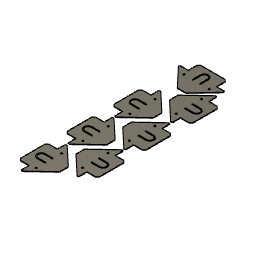
MagneticClampHanger v1 (Autodesk Fusion 360 design; units mm, degrees)
Autodesk Fusion 360 part; units mm, degrees
sketch "Sketch1" plane through (0, 0, 0) normal (0, 1, 0) x (1, 0, 0)
  line L0 (0, 0) -> (92.202, 0)
  line L1 (0, 0) -> (0, 34.29)
  line L2 (92.202, 0) -> (92.202, 34.29)
  line L3 (0, 34.29) -> (-31.75, 34.29)
  line L4 (92.202, 34.29) -> (123.952, 34.29)
  line L5 (46.101, 0) -> (46.101, 101.981) construction
  line L6 (46.101, 101.981) -> (60.071, 101.981) construction
  line L7 (60.071, 101.981) -> (123.952, 34.29)
  line L8 (60.071, 101.981) -> (32.131, 101.981)
  line L9 (32.131, 101.981) -> (-31.75, 34.29)
  line L10 (46.101, 0) -> (46.101, 31.75) construction
  line L11 (46.101, 101.981) -> (46.101, 60.833) construction
  line L12 (46.101, 60.833) -> (46.101, 46.2915) construction
  circle A0 centre (46.101, 46.2915) radius 14.5415 construction
  line L13 (-6.604, -6.604) -> (-6.604, 27.686)
  line L14 (-6.604, 27.686) -> (-47.0627, 27.686)
  line L15 (29.2829, 108.585) -> (-47.0627, 27.686)
  line L16 (62.9191, 108.585) -> (29.2829, 108.585)
  line L17 (62.9191, 108.585) -> (139.2647, 27.686)
  line L18 (98.806, 27.686) -> (139.2647, 27.686)
  line L19 (98.806, -6.604) -> (98.806, 27.686)
  line L20 (-6.604, -6.604) -> (98.806, -6.604)
  line L21 (58.6943, 53.5623) -> (33.5077, 53.5623) construction
  line L22 (33.5077, 53.5623) -> (35.0952, 53.5623)
  line L23 (58.6943, 53.5623) -> (57.1068, 53.5623)
  line L24 (35.0952, 53.5623) -> (35.0952, 28.1623)
  line L25 (57.1068, 53.5623) -> (57.1068, 28.1623)
  arc A1 (35.0952, 28.1623) -> (57.1068, 28.1623) centre (46.101, 28.1623) ccw
  line L26 (33.5077, 51.9748) -> (33.5077, 28.1623)
  arc A2 (33.5077, 28.1623) -> (58.6943, 28.1623) centre (46.101, 28.1623) ccw
  line L27 (58.6943, 51.9748) -> (58.6943, 28.1623)
  line L28 (33.5077, 51.9748) -> (33.5077, 53.5623)
  line L29 (58.6943, 51.9748) -> (58.6943, 53.5623)
  dimension "d1" = 92.202
  dimension "d2" = 34.29
  dimension "d3" = 34.29
  dimension "d4" = 31.75
  dimension "d5" = 31.75
  dimension "d6" = 101.981
  dimension "d7" = 13.97
  dimension "d8" = 27.94
  dimension "d9" = 31.75
  dimension "d10" = 41.148
  dimension "d11" = 14.5415
  dimension "d12" = 6.604
  dimension "d13" = 1.5875
  dimension "d14" = 1.5875
  dimension "d15" = 25.4
  dimension "d16" = 25.4
  dimension "d17" = 1.5875
  constraint coincident L0.start L1.start
  constraint horizontal L0
  constraint perpendicular L0 L1
  constraint perpendicular L0 L2
  constraint perpendicular L1 L3
  constraint perpendicular L2 L4
  constraint midpoint L0 L5.start
  constraint perpendicular L0 L5
  constraint perpendicular L5 L6
  constraint perpendicular L5 L8
  constraint perpendicular L0 L10
  constraint perpendicular L8 L11
  constraint perpendicular L4 L12
  constraint coincident L12.end A0.centre
  constraint coincident L10.end A0
  constraint coincident A0 L21.start
  constraint coincident A0 L21.end
  constraint perpendicular L5 L21
  constraint parallel L21 L22
  constraint parallel L21 L23
  constraint perpendicular L21 L24
  constraint perpendicular L21 L25
  constraint tangent L25 A1
  constraint perpendicular L21 L28
  constraint perpendicular L21 L29
  measures "d1" distance of L0.start L0.end
  measures "d2" distance of L0.start L1.end
  measures "d3" distance of L0.end L2.end
  measures "d4" distance of L1.end L3.end
  measures "d5" distance of L2.end L4.end
  measures "d6" distance of L5.start L5.end
  measures "d7" distance of L5.end L6.end
  measures "d8" distance of L6.end L8.end
  measures "d9" distance of L5.start L10.end
  measures "d10" distance of L5.end L11.end
  measures "d11" distance of L11.end L12.end
  measures "d13" distance of L21.end L22.end
  measures "d14" distance of L21.start L23.end
  measures "d15" distance of L22.end L24.end
  measures "d16" distance of L23.end L25.end
extrude "Extrude1" add sketch "Sketch1" along normal blind 1.5875 contours L0 L1 L2 L3 L4 L7 L8 L9 makes body 1
fillet "Fillet1" radius 0.7937 4 edges at (33.5077, 0.7937, -53.5623) (35.0952, 0.7937, -53.5623) (58.6943, 0.7937, -53.5623) (57.1068, 0.7937, -53.5623) on bodies 1
chamfer "Chamfer1" distance 6.35 angle 45 4 edges at (92.202, 0.7937, 0) (0, 0.7937, 0) (-31.75, 0.7937, -34.29) (123.952, 0.7937, -34.29) on bodies 1
sketch "Sketch2" plane through (0, 1.5875, 0) normal (0, 1, 0) x (-1, 0, 0)
  line L0 (-117.602, -34.29) -> (-119.5937, -38.9082)
  line L1 (-119.5937, -38.9082) -> (-60.071, -101.981)
  line L2 (-60.071, -101.981) -> (-32.131, -101.981)
  line L3 (-32.131, -101.981) -> (27.3917, -38.9082)
  line L4 (27.3917, -38.9082) -> (25.4, -34.29)
  line L5 (25.4, -34.29) -> (0, -34.29)
  line L6 (0, -34.29) -> (0, -6.35)
  line L7 (0, -6.35) -> (-6.35, 0)
  line L8 (-6.35, 0) -> (-85.852, 0)
  line L9 (-85.852, 0) -> (-92.202, -6.35)
  line L10 (-92.202, -6.35) -> (-92.202, -34.29)
  line L11 (-92.202, -34.29) -> (-117.602, -34.29)
  line L12 (-33.5077, -28.1623) -> (-33.5077, -52.7685)
  arc A0 (-35.0952, -52.7685) -> (-33.5077, -52.7685) centre (-34.3014, -52.7685) ccw
  line L13 (-35.0952, -52.7685) -> (-35.0952, -28.1623)
  arc A1 (-35.0952, -28.1623) -> (-57.1068, -28.1623) centre (-46.101, -28.1623) ccw
  line L14 (-57.1068, -28.1623) -> (-57.1068, -52.7685)
  arc A2 (-58.6943, -52.7685) -> (-57.1068, -52.7685) centre (-57.9006, -52.7685) ccw
  line L15 (-58.6943, -52.7685) -> (-58.6943, -28.1623)
  arc A3 (-33.5077, -28.1623) -> (-58.6943, -28.1623) centre (-46.101, -28.1623) ccw
  line L16 (27.3917, -38.9082) -> (14.3169, -52.7629) construction
  line L17 (-119.5937, -38.9082) -> (-106.5189, -52.7629) construction
  line L18 (14.3169, -52.7629) -> (-4.7331, -52.7629) construction
  line L19 (-106.5189, -52.7629) -> (-87.4689, -52.7629) construction
  circle A4 centre (-4.7331, -52.7629) radius 2.54
  circle A5 centre (-87.4689, -52.7629) radius 2.54
  dimension "d23" = 19.05
  dimension "d24" = 19.05
  dimension "d25" = 19.05
  dimension "d26" = 19.05
  dimension "d27" = 5.08
  dimension "d28" = 5.08
  constraint coincident L3.end L4.start
  constraint parallel L3 L16
  constraint coincident L0.end L1.start
  constraint parallel L1 L17
  constraint horizontal L18
  constraint horizontal L19
  constraint coincident L18.end A4.centre
  constraint coincident L19.end A5.centre
  measures "d23" distance of L3.end L16.end
  measures "d24" distance of L0.end L17.end
  measures "d25" distance of L16.end L18.end
  measures "d26" distance of L17.end L19.end
  measures "d27" diameter of A4
  measures "d28" diameter of A5
extrude "Extrude2" cut sketch "Sketch2" against normal up to surface (1.5875 mm away) contours A4 | A5 bodies 1
copy_body "Body->Comp1" bodies 1 removing the originals makes body 2 in component "Component"
sketch "Sketch4" plane through (0, 1.5875, 0) normal (0, 1, 0) x (-1, 0, 0)
  circle A0 centre (-27.5724, -119.0093) radius 2.54
  circle A1 centre (-27.5724, -36.2735) radius 2.54
  line L0 (-9.0996, -6.1404) -> (-13.7178, -4.1487)
  line L1 (-13.7178, -4.1487) -> (-76.7906, -63.6714)
  line L2 (-76.7906, -63.6714) -> (-76.7906, -91.6114)
  line L3 (-76.7906, -91.6114) -> (-13.7178, -151.1342)
  line L4 (-13.7178, -151.1342) -> (-9.0996, -149.1424)
  line L5 (-9.0996, -149.1424) -> (-9.0996, -123.7424)
  line L6 (-9.0996, -123.7424) -> (18.8404, -123.7424)
  line L7 (18.8404, -123.7424) -> (25.1904, -117.3924)
  line L8 (25.1904, -117.3924) -> (25.1904, -37.8904)
  line L9 (25.1904, -37.8904) -> (18.8404, -31.5404)
  line L10 (18.8404, -31.5404) -> (-9.0996, -31.5404)
  line L11 (-9.0996, -31.5404) -> (-9.0996, -6.1404)
  line L12 (-2.9718, -90.2347) -> (-27.5781, -90.2347)
  arc A2 (-27.5781, -88.6472) -> (-27.5781, -90.2347) centre (-27.5781, -89.441) ccw
  line L13 (-27.5781, -88.6472) -> (-2.9718, -88.6472)
  arc A3 (-2.9718, -88.6472) -> (-2.9718, -66.6356) centre (-2.9718, -77.6414) ccw
  line L14 (-2.9718, -66.6356) -> (-27.5781, -66.6356)
  arc A4 (-27.5781, -65.0481) -> (-27.5781, -66.6356) centre (-27.5781, -65.8419) ccw
  line L15 (-27.5781, -65.0481) -> (-2.9718, -65.0481)
  arc A5 (-2.9718, -90.2347) -> (-2.9718, -65.0481) centre (-2.9718, -77.6414) ccw
  line L16 (33.02, 0) -> (-170.18, 0)
  line L17 (-170.18, 0) -> (-170.18, -609.6)
  line L18 (-170.18, -609.6) -> (33.02, -609.6)
  line L19 (33.02, -609.6) -> (33.02, 0)
  dimension "d33" = 203.2
  constraint horizontal L16
  constraint vertical L17
  constraint horizontal L18
  constraint vertical L19
  measures "d33" distance of L16.start L16.end
extrude "Extrude1'" add sketch "Sketch4" against normal blind 1.5875 separate body contours A0 | A1 | L0 L1 L2 L3 L4 L5 L6 L7 L8 L9 L10 L11 | L12 A2 L13 A3 L14 A4 L15 A5 | L16 L17 L18 L19 makes body 3 in component "Component'"
move_face "OffsetFaces1" offset -0.635 3 faces at (58.6943, 0.5292, -44.5665) (55.748, 0.5292, -20.0674) (33.5077, 0.5292, -36.3644) on bodies 2 in component "Component"
sketch "Sketch5" plane through (0, 1.5875, 0) normal (0, 1, 0) x (-1, 0, 0)
  circle A0 centre (-102.7296, -417.2735) radius 2.54
  circle A1 centre (-102.7296, -500.0093) radius 2.54
  line L0 (-121.2024, -530.1424) -> (-116.5842, -532.1342)
  line L1 (-116.5842, -532.1342) -> (-53.5114, -472.6114)
  line L2 (-53.5114, -472.6114) -> (-53.5114, -444.6714)
  line L3 (-53.5114, -444.6714) -> (-116.5842, -385.1487)
  line L4 (-116.5842, -385.1487) -> (-121.2024, -387.1404)
  line L5 (-121.2024, -387.1404) -> (-121.2024, -412.5404)
  line L6 (-121.2024, -412.5404) -> (-149.1424, -412.5404)
  line L7 (-149.1424, -412.5404) -> (-155.4924, -418.8904)
  line L8 (-155.4924, -418.8904) -> (-155.4924, -498.3924)
  line L9 (-155.4924, -498.3924) -> (-149.1424, -504.7424)
  line L10 (-149.1424, -504.7424) -> (-121.2024, -504.7424)
  line L11 (-121.2024, -504.7424) -> (-121.2024, -530.1424)
  line L12 (-127.3302, -445.4131) -> (-102.7239, -445.4131)
  arc A2 (-102.7239, -448.2706) -> (-102.7239, -445.4131) centre (-102.7239, -446.8419) ccw
  line L13 (-102.7239, -448.2706) -> (-127.3302, -448.2706)
  arc A3 (-127.3302, -448.2706) -> (-127.3302, -469.0122) centre (-127.3302, -458.6414) ccw
  line L14 (-127.3302, -469.0122) -> (-102.7239, -469.0122)
  arc A4 (-102.7239, -471.8697) -> (-102.7239, -469.0122) centre (-102.7239, -470.441) ccw
  line L15 (-102.7239, -471.8697) -> (-127.3302, -471.8697)
  arc A5 (-127.3302, -445.4131) -> (-127.3302, -471.8697) centre (-127.3302, -458.6414) ccw
component "Component" placed x (0, 0, 1) y (0, 1, 0) z (-1, 0, 0) at (-25.1904, 0, -123.7424)
component "Component" placed x (0, 0, -1) y (0, 1, 0) z (1, 0, 0) at (155.4924, 0, -107.7404)
component "Component" placed x (0, 0, 1) y (0, 1, 0) z (-1, 0, 0) at (-25.1904, 0, -276.1424)
component "Component" placed x (0, 0, -1) y (0, 1, 0) z (1, 0, 0) at (155.4924, 0, -412.5404)
component "Component" placed x (0, 0, -1) y (0, 1, 0) z (1, 0, 0) at (155.4924, 0, -260.1404)
component "Component" placed x (0, 0, 1) y (0, 1, 0) z (-1, 0, 0) at (-25.1904, 0, -428.5424)
component "Component" placed x (-1, 0, 0) y (0, 1, 0) z (0, 0, -1) at (92.202, 0, -593.4329)
component "Component'" placed x (1, 0, 0) y (0, 1, 0) z (0, 0, 1) at (0, 0, 0)
equation "d7 = ( 1.1 / 2 ) * 1 in"
equation "d11 = ( 1.145 / 2 ) * 1 in"
equation "d13 = ( 1 / 16 ) * 1 in"
equation "d14 = ( 1 / 16 ) * 1 in"
equation "d17 = ( 1 / 16 ) * 1 in"
equation "d18 = ( 1 / 16 ) * 1 in"
equation "d21 = ( 1 / 32 ) * 1 in"
equation "d34 = ( -1 / 16 ) * 1 in"
